Autodesk Fusion 360 part; units mm, degrees
(part 2 of 4)
sketch "스케치3" plane through (0, 0, 0) normal (0, 0, 1) x (1, 0, 0)
  line L0 (5.08, 57.675) -> (15.18, 57.675)
  line L1 (15.18, 57.675) -> (15.18, 47.575)
  line L2 (15.18, 47.575) -> (5.08, 47.575)
  line L3 (5.08, 47.575) -> (5.08, 57.675)
  line L4 (10.13, 57.675) -> (10.13, 47.575) construction
  line L5 (15.18, 52.625) -> (5.08, 52.625) construction
  line L6 (5.08, 53.975) -> (5.08, 51.275) construction
  line L7 (15.18, 53.975) -> (15.18, 51.275) construction
  line L8 (8.78, 57.675) -> (11.48, 57.675) construction
  line L9 (8.78, 47.575) -> (11.48, 47.575) construction
  line L10 (8.78, 57.675) -> (9.13, 56.625)
  line L11 (9.13, 56.625) -> (11.13, 56.625)
  line L12 (11.13, 56.625) -> (11.48, 57.675)
  line L13 (11.48, 47.575) -> (11.13, 48.625)
  line L14 (11.13, 48.625) -> (9.13, 48.625)
  line L15 (9.13, 48.625) -> (8.78, 47.575)
  line L16 (5.08, 51.275) -> (6.13, 51.625)
  line L17 (6.13, 51.625) -> (6.13, 53.625)
  line L18 (6.13, 53.625) -> (5.08, 53.975)
  line L19 (15.18, 53.975) -> (14.13, 53.625)
  line L20 (14.13, 53.625) -> (14.13, 51.625)
  line L21 (14.13, 51.625) -> (15.18, 51.275)
  line L22 (6.13, 53.625) -> (5.08, 53.625) construction
  line L23 (11.13, 56.625) -> (11.13, 57.675) construction
  line L24 (9.13, 48.625) -> (9.13, 47.575) construction
  line L25 (14.13, 51.625) -> (15.18, 51.625) construction
  circle A0 centre (10.13, 52.625) radius 5.05 construction
  line L26 (19.78, 51.625) -> (19.78, 53.625)
  line L27 (18.73, 53.975) -> (18.73, 51.275)
  line L28 (22.43, 47.575) -> (25.13, 47.575)
  line L29 (19.78, 53.625) -> (18.73, 53.625) construction
  line L30 (27.78, 51.625) -> (28.83, 51.275)
  line L31 (18.73, 51.275) -> (19.78, 51.625)
  line L32 (24.78, 56.625) -> (24.78, 57.675) construction
  line L33 (27.78, 53.625) -> (27.78, 51.625)
  line L34 (24.78, 48.625) -> (22.78, 48.625)
  line L35 (28.83, 53.975) -> (27.78, 53.625)
  line L36 (24.78, 56.625) -> (25.13, 57.675)
  line L37 (22.43, 57.675) -> (22.78, 56.625)
  line L38 (28.83, 52.625) -> (18.73, 52.625) construction
  line L39 (28.83, 53.975) -> (28.83, 51.275)
  line L40 (22.78, 48.625) -> (22.43, 47.575)
  line L41 (22.78, 48.625) -> (22.78, 47.575) construction
  line L42 (27.78, 51.625) -> (28.83, 51.625) construction
  line L43 (22.43, 57.675) -> (25.13, 57.675)
  line L44 (25.13, 47.575) -> (24.78, 48.625)
  line L45 (19.78, 53.625) -> (18.73, 53.975)
  line L46 (23.78, 57.675) -> (23.78, 47.575) construction
  line L47 (22.78, 56.625) -> (24.78, 56.625)
  circle A1 centre (23.78, 52.625) radius 5.05 construction
  line L48 (39.07, 56.625) -> (39.42, 57.675)
  line L49 (37.07, 48.625) -> (37.07, 47.575) construction
  line L50 (33.02, 53.975) -> (33.02, 51.275)
  line L51 (36.72, 57.675) -> (37.07, 56.625)
  line L52 (36.72, 57.675) -> (39.42, 57.675)
  line L53 (38.07, 57.675) -> (38.07, 47.575) construction
  line L54 (34.07, 51.625) -> (34.07, 53.625)
  line L55 (37.07, 48.625) -> (36.72, 47.575)
  line L56 (37.07, 56.625) -> (39.07, 56.625)
  line L57 (34.07, 53.625) -> (33.02, 53.975)
  line L58 (33.02, 51.275) -> (34.07, 51.625)
  line L59 (39.07, 48.625) -> (37.07, 48.625)
  line L60 (39.42, 47.575) -> (39.07, 48.625)
  line L61 (36.72, 47.575) -> (39.42, 47.575)
  line L62 (34.07, 53.625) -> (33.02, 53.625) construction
  line L63 (39.07, 56.625) -> (39.07, 57.675) construction
  line L64 (42.07, 51.625) -> (43.12, 51.625) construction
  line L65 (43.12, 52.625) -> (33.02, 52.625) construction
  line L66 (42.07, 51.625) -> (43.12, 51.275)
  line L67 (43.12, 53.975) -> (43.12, 51.275)
  circle A2 centre (38.07, 52.625) radius 5.05 construction
  line L68 (42.07, 53.625) -> (42.07, 51.625)
  line L69 (43.12, 53.975) -> (42.07, 53.625)
  line L70 (53.04, 56.625) -> (53.39, 57.675)
  line L71 (51.04, 48.625) -> (51.04, 47.575) construction
  line L72 (46.99, 53.975) -> (46.99, 51.275)
  line L73 (50.69, 57.675) -> (51.04, 56.625)
  line L74 (50.69, 57.675) -> (53.39, 57.675)
  line L75 (52.04, 57.675) -> (52.04, 47.575) construction
  line L76 (48.04, 51.625) -> (48.04, 53.625)
  line L77 (51.04, 48.625) -> (50.69, 47.575)
  line L78 (51.04, 56.625) -> (53.04, 56.625)
  line L79 (48.04, 53.625) -> (46.99, 53.975)
  line L80 (46.99, 51.275) -> (48.04, 51.625)
  line L81 (53.04, 48.625) -> (51.04, 48.625)
  line L82 (53.39, 47.575) -> (53.04, 48.625)
  line L83 (50.69, 47.575) -> (53.39, 47.575)
  line L84 (48.04, 53.625) -> (46.99, 53.625) construction
  line L85 (53.04, 56.625) -> (53.04, 57.675) construction
  line L86 (56.04, 51.625) -> (57.09, 51.625) construction
  line L87 (57.09, 52.625) -> (46.99, 52.625) construction
  line L88 (56.04, 51.625) -> (57.09, 51.275)
  line L89 (57.09, 53.975) -> (57.09, 51.275)
  circle A3 centre (52.04, 52.625) radius 5.05 construction
  line L90 (56.04, 53.625) -> (56.04, 51.625)
  line L91 (57.09, 53.975) -> (56.04, 53.625)
  line L92 (67.01, 56.625) -> (67.36, 57.675)
  line L93 (65.01, 48.625) -> (65.01, 47.575) construction
  line L94 (60.96, 53.975) -> (60.96, 51.275)
  line L95 (64.66, 57.675) -> (65.01, 56.625)
  line L96 (64.66, 57.675) -> (67.36, 57.675)
  line L97 (66.01, 57.675) -> (66.01, 47.575) construction
  line L98 (62.01, 51.625) -> (62.01, 53.625)
  line L99 (65.01, 48.625) -> (64.66, 47.575)
  line L100 (65.01, 56.625) -> (67.01, 56.625)
  line L101 (62.01, 53.625) -> (60.96, 53.975)
  line L102 (60.96, 51.275) -> (62.01, 51.625)
  line L103 (67.01, 48.625) -> (65.01, 48.625)
  line L104 (67.36, 47.575) -> (67.01, 48.625)
  line L105 (64.66, 47.575) -> (67.36, 47.575)
  line L106 (62.01, 53.625) -> (60.96, 53.625) construction
  line L107 (67.01, 56.625) -> (67.01, 57.675) construction
  line L108 (70.01, 51.625) -> (71.06, 51.625) construction
  line L109 (71.06, 52.625) -> (60.96, 52.625) construction
  line L110 (70.01, 51.625) -> (71.06, 51.275)
  line L111 (71.06, 53.975) -> (71.06, 51.275)
  circle A4 centre (66.01, 52.625) radius 5.05 construction
  line L112 (70.01, 53.625) -> (70.01, 51.625)
  line L113 (71.06, 53.975) -> (70.01, 53.625)
  line L114 (80.98, 56.625) -> (81.33, 57.675)
  line L115 (78.98, 48.625) -> (78.98, 47.575) construction
  line L116 (74.93, 53.975) -> (74.93, 51.275)
  line L117 (78.63, 57.675) -> (78.98, 56.625)
  line L118 (78.63, 57.675) -> (81.33, 57.675)
  line L119 (79.98, 57.675) -> (79.98, 47.575) construction
  line L120 (75.98, 51.625) -> (75.98, 53.625)
  line L121 (78.98, 48.625) -> (78.63, 47.575)
  line L122 (78.98, 56.625) -> (80.98, 56.625)
  line L123 (75.98, 53.625) -> (74.93, 53.975)
  line L124 (74.93, 51.275) -> (75.98, 51.625)
  line L125 (80.98, 48.625) -> (78.98, 48.625)
  line L126 (81.33, 47.575) -> (80.98, 48.625)
  line L127 (78.63, 47.575) -> (81.33, 47.575)
  line L128 (75.98, 53.625) -> (74.93, 53.625) construction
  line L129 (80.98, 56.625) -> (80.98, 57.675) construction
  line L130 (83.98, 51.625) -> (85.03, 51.625) construction
  line L131 (85.03, 52.625) -> (74.93, 52.625) construction
  line L132 (83.98, 51.625) -> (85.03, 51.275)
  line L133 (85.03, 53.975) -> (85.03, 51.275)
  circle A5 centre (79.98, 52.625) radius 5.05 construction
  line L134 (83.98, 53.625) -> (83.98, 51.625)
  line L135 (85.03, 53.975) -> (83.98, 53.625)
  line L136 (94.95, 56.625) -> (95.3, 57.675)
  line L137 (92.95, 48.625) -> (92.95, 47.575) construction
  line L138 (88.9, 53.975) -> (88.9, 51.275)
  line L139 (92.6, 57.675) -> (92.95, 56.625)
  line L140 (92.6, 57.675) -> (95.3, 57.675)
  line L141 (93.95, 57.675) -> (93.95, 47.575) construction
  line L142 (89.95, 51.625) -> (89.95, 53.625)
  line L143 (92.95, 48.625) -> (92.6, 47.575)
  line L144 (92.95, 56.625) -> (94.95, 56.625)
  line L145 (89.95, 53.625) -> (88.9, 53.975)
  line L146 (88.9, 51.275) -> (89.95, 51.625)
  line L147 (94.95, 48.625) -> (92.95, 48.625)
  line L148 (95.3, 47.575) -> (94.95, 48.625)
  line L149 (92.6, 47.575) -> (95.3, 47.575)
  line L150 (89.95, 53.625) -> (88.9, 53.625) construction
  line L151 (94.95, 56.625) -> (94.95, 57.675) construction
  line L152 (97.95, 51.625) -> (99, 51.625) construction
  line L153 (99, 52.625) -> (88.9, 52.625) construction
  line L154 (97.95, 51.625) -> (99, 51.275)
  line L155 (99, 53.975) -> (99, 51.275)
  circle A6 centre (93.95, 52.625) radius 5.05 construction
  line L156 (97.95, 53.625) -> (97.95, 51.625)
  line L157 (99, 53.975) -> (97.95, 53.625)
  line L158 (108.92, 56.625) -> (109.27, 57.675)
  line L159 (106.92, 48.625) -> (106.92, 47.575) construction
  line L160 (102.87, 53.975) -> (102.87, 51.275)
  line L161 (106.57, 57.675) -> (106.92, 56.625)
  line L162 (106.57, 57.675) -> (109.27, 57.675)
  line L163 (107.92, 57.675) -> (107.92, 47.575) construction
  line L164 (103.92, 51.625) -> (103.92, 53.625)
  line L165 (106.92, 48.625) -> (106.57, 47.575)
  line L166 (106.92, 56.625) -> (108.92, 56.625)
  line L167 (103.92, 53.625) -> (102.87, 53.975)
  line L168 (102.87, 51.275) -> (103.92, 51.625)
  line L169 (108.92, 48.625) -> (106.92, 48.625)
  line L170 (109.27, 47.575) -> (108.92, 48.625)
  line L171 (106.57, 47.575) -> (109.27, 47.575)
  line L172 (103.92, 53.625) -> (102.87, 53.625) construction
  line L173 (108.92, 56.625) -> (108.92, 57.675) construction
  line L174 (111.92, 51.625) -> (112.97, 51.625) construction
  line L175 (112.97, 52.625) -> (102.87, 52.625) construction
  line L176 (111.92, 51.625) -> (112.97, 51.275)
  line L177 (112.97, 53.975) -> (112.97, 51.275)
  circle A7 centre (107.92, 52.625) radius 5.05 construction
  line L178 (111.92, 53.625) -> (111.92, 51.625)
  line L179 (112.97, 53.975) -> (111.92, 53.625)
  line L180 (122.89, 56.625) -> (123.24, 57.675)
  line L181 (120.89, 48.625) -> (120.89, 47.575) construction
  line L182 (116.84, 53.975) -> (116.84, 51.275)
  line L183 (120.54, 57.675) -> (120.89, 56.625)
  line L184 (120.54, 57.675) -> (123.24, 57.675)
  line L185 (121.89, 57.675) -> (121.89, 47.575) construction
  line L186 (117.89, 51.625) -> (117.89, 53.625)
  line L187 (120.89, 48.625) -> (120.54, 47.575)
  line L188 (120.89, 56.625) -> (122.89, 56.625)
  line L189 (117.89, 53.625) -> (116.84, 53.975)
  line L190 (116.84, 51.275) -> (117.89, 51.625)
  line L191 (122.89, 48.625) -> (120.89, 48.625)
  line L192 (123.24, 47.575) -> (122.89, 48.625)
  line L193 (120.54, 47.575) -> (123.24, 47.575)
  line L194 (117.89, 53.625) -> (116.84, 53.625) construction
  line L195 (122.89, 56.625) -> (122.89, 57.675) construction
  line L196 (125.89, 51.625) -> (126.94, 51.625) construction
  line L197 (126.94, 52.625) -> (116.84, 52.625) construction
  line L198 (125.89, 51.625) -> (126.94, 51.275)
  line L199 (126.94, 53.975) -> (126.94, 51.275)
  circle A8 centre (121.89, 52.625) radius 5.05 construction
  line L200 (125.89, 53.625) -> (125.89, 51.625)
  line L201 (126.94, 53.975) -> (125.89, 53.625)
  line L202 (136.86, 56.625) -> (137.21, 57.675)
  line L203 (134.86, 48.625) -> (134.86, 47.575) construction
  line L204 (130.81, 53.975) -> (130.81, 51.275)
  line L205 (134.51, 57.675) -> (134.86, 56.625)
  line L206 (134.51, 57.675) -> (137.21, 57.675)
  line L207 (135.86, 57.675) -> (135.86, 47.575) construction
  line L208 (131.86, 51.625) -> (131.86, 53.625)
  line L209 (134.86, 48.625) -> (134.51, 47.575)
  line L210 (134.86, 56.625) -> (136.86, 56.625)
  line L211 (131.86, 53.625) -> (130.81, 53.975)
  line L212 (130.81, 51.275) -> (131.86, 51.625)
  line L213 (136.86, 48.625) -> (134.86, 48.625)
  line L214 (137.21, 47.575) -> (136.86, 48.625)
  line L215 (134.51, 47.575) -> (137.21, 47.575)
  line L216 (131.86, 53.625) -> (130.81, 53.625) construction
  line L217 (136.86, 56.625) -> (136.86, 57.675) construction
  line L218 (139.86, 51.625) -> (140.91, 51.625) construction
  line L219 (140.91, 52.625) -> (130.81, 52.625) construction
  line L220 (139.86, 51.625) -> (140.91, 51.275)
  line L221 (140.91, 53.975) -> (140.91, 51.275)
  circle A9 centre (135.86, 52.625) radius 5.05 construction
  line L222 (139.86, 53.625) -> (139.86, 51.625)
  line L223 (140.91, 53.975) -> (139.86, 53.625)
  circle A10 centre (30.453, 38.655) radius 5.05 construction
  line L224 (29.103, 43.705) -> (29.453, 42.655)
  line L225 (34.453, 37.655) -> (35.503, 37.655) construction
  line L226 (34.453, 39.655) -> (34.453, 37.655)
  line L227 (25.403, 40.005) -> (25.403, 37.305)
  line L228 (31.453, 34.655) -> (29.453, 34.655)
  line L229 (26.453, 37.655) -> (26.453, 39.655)
  line L230 (31.453, 42.655) -> (31.453, 43.705) construction
  line L231 (25.403, 37.305) -> (26.453, 37.655)
  line L232 (31.803, 33.605) -> (31.453, 34.655)
  line L233 (29.453, 34.655) -> (29.453, 33.605) construction
  line L234 (35.503, 40.005) -> (35.503, 37.305)
  line L235 (29.103, 43.705) -> (31.803, 43.705)
  line L236 (35.503, 38.655) -> (25.403, 38.655) construction
  line L237 (29.453, 34.655) -> (29.103, 33.605)
  line L238 (30.453, 43.705) -> (30.453, 33.605) construction
  line L239 (34.453, 37.655) -> (35.503, 37.305)
  line L240 (35.503, 40.005) -> (34.453, 39.655)
  line L241 (29.103, 33.605) -> (31.803, 33.605)
  line L242 (31.453, 42.655) -> (31.803, 43.705)
  line L243 (29.453, 42.655) -> (31.453, 42.655)
  line L244 (26.453, 39.655) -> (25.403, 40.005)
  line L245 (26.453, 39.655) -> (25.403, 39.655) construction
  circle A11 centre (44.423, 38.655) radius 5.05 construction
  line L246 (43.073, 43.705) -> (43.423, 42.655)
  line L247 (48.423, 37.655) -> (49.473, 37.655) construction
  line L248 (48.423, 39.655) -> (48.423, 37.655)
  line L249 (39.373, 40.005) -> (39.373, 37.305)
  line L250 (45.423, 34.655) -> (43.423, 34.655)
  line L251 (40.423, 37.655) -> (40.423, 39.655)
  line L252 (45.423, 42.655) -> (45.423, 43.705) construction
  line L253 (39.373, 37.305) -> (40.423, 37.655)
  line L254 (45.773, 33.605) -> (45.423, 34.655)
  line L255 (43.423, 34.655) -> (43.423, 33.605) construction
  line L256 (49.473, 40.005) -> (49.473, 37.305)
  line L257 (43.073, 43.705) -> (45.773, 43.705)
  line L258 (49.473, 38.655) -> (39.373, 38.655) construction
  line L259 (43.423, 34.655) -> (43.073, 33.605)
  line L260 (44.423, 43.705) -> (44.423, 33.605) construction
  line L261 (48.423, 37.655) -> (49.473, 37.305)
  line L262 (49.473, 40.005) -> (48.423, 39.655)
  line L263 (43.073, 33.605) -> (45.773, 33.605)
  line L264 (45.423, 42.655) -> (45.773, 43.705)
  line L265 (43.423, 42.655) -> (45.423, 42.655)
  line L266 (40.423, 39.655) -> (39.373, 40.005)
  line L267 (40.423, 39.655) -> (39.373, 39.655) construction
  circle A12 centre (58.393, 38.655) radius 5.05 construction
  line L268 (57.043, 43.705) -> (57.393, 42.655)
  line L269 (62.393, 37.655) -> (63.443, 37.655) construction
  line L270 (62.393, 39.655) -> (62.393, 37.655)
  line L271 (53.343, 40.005) -> (53.343, 37.305)
  line L272 (59.393, 34.655) -> (57.393, 34.655)
  line L273 (54.393, 37.655) -> (54.393, 39.655)
  line L274 (59.393, 42.655) -> (59.393, 43.705) construction
  line L275 (53.343, 37.305) -> (54.393, 37.655)
  line L276 (59.743, 33.605) -> (59.393, 34.655)
  line L277 (57.393, 34.655) -> (57.393, 33.605) construction
  line L278 (63.443, 40.005) -> (63.443, 37.305)
  line L279 (57.043, 43.705) -> (59.743, 43.705)
  line L280 (63.443, 38.655) -> (53.343, 38.655) construction
  line L281 (57.393, 34.655) -> (57.043, 33.605)
  line L282 (58.393, 43.705) -> (58.393, 33.605) construction
  line L283 (62.393, 37.655) -> (63.443, 37.305)
  line L284 (63.443, 40.005) -> (62.393, 39.655)
  line L285 (57.043, 33.605) -> (59.743, 33.605)
  line L286 (59.393, 42.655) -> (59.743, 43.705)
  line L287 (57.393, 42.655) -> (59.393, 42.655)
  line L288 (54.393, 39.655) -> (53.343, 40.005)
  line L289 (54.393, 39.655) -> (53.343, 39.655) construction
  circle A13 centre (72.363, 38.655) radius 5.05 construction
  line L290 (71.013, 43.705) -> (71.363, 42.655)
  line L291 (76.363, 37.655) -> (77.413, 37.655) construction
  line L292 (76.363, 39.655) -> (76.363, 37.655)
  line L293 (67.313, 40.005) -> (67.313, 37.305)
  line L294 (73.363, 34.655) -> (71.363, 34.655)
  line L295 (68.363, 37.655) -> (68.363, 39.655)
  line L296 (73.363, 42.655) -> (73.363, 43.705) construction
  line L297 (67.313, 37.305) -> (68.363, 37.655)
  line L298 (73.713, 33.605) -> (73.363, 34.655)
  line L299 (71.363, 34.655) -> (71.363, 33.605) construction
  line L300 (77.413, 40.005) -> (77.413, 37.305)
  line L301 (71.013, 43.705) -> (73.713, 43.705)
  line L302 (77.413, 38.655) -> (67.313, 38.655) construction
  line L303 (71.363, 34.655) -> (71.013, 33.605)
  line L304 (72.363, 43.705) -> (72.363, 33.605) construction
  line L305 (76.363, 37.655) -> (77.413, 37.305)
  line L306 (77.413, 40.005) -> (76.363, 39.655)
  line L307 (71.013, 33.605) -> (73.713, 33.605)
  line L308 (73.363, 42.655) -> (73.713, 43.705)
  line L309 (71.363, 42.655) -> (73.363, 42.655)
  line L310 (68.363, 39.655) -> (67.313, 40.005)
  line L311 (68.363, 39.655) -> (67.313, 39.655) construction
  circle A14 centre (16.483, 38.655) radius 5.05 construction
  line L312 (15.133, 43.705) -> (15.483, 42.655)
  line L313 (20.483, 37.655) -> (21.533, 37.655) construction
  line L314 (20.483, 39.655) -> (20.483, 37.655)
  line L315 (11.433, 40.005) -> (11.433, 37.305)
  line L316 (17.483, 34.655) -> (15.483, 34.655)
  line L317 (12.483, 37.655) -> (12.483, 39.655)
  line L318 (17.483, 42.655) -> (17.483, 43.705) construction
  line L319 (11.433, 37.305) -> (12.483, 37.655)
  line L320 (17.833, 33.605) -> (17.483, 34.655)
  line L321 (15.483, 34.655) -> (15.483, 33.605) construction
  line L322 (21.533, 40.005) -> (21.533, 37.305)
  line L323 (15.133, 43.705) -> (17.833, 43.705)
  line L324 (21.533, 38.655) -> (11.433, 38.655) construction
  line L325 (15.483, 34.655) -> (15.133, 33.605)
  line L326 (16.483, 43.705) -> (16.483, 33.605) construction
  line L327 (20.483, 37.655) -> (21.533, 37.305)
  line L328 (21.533, 40.005) -> (20.483, 39.655)
  line L329 (15.133, 33.605) -> (17.833, 33.605)
  line L330 (17.483, 42.655) -> (17.833, 43.705)
  line L331 (15.483, 42.655) -> (17.483, 42.655)
  line L332 (12.483, 39.655) -> (11.433, 40.005)
  line L333 (12.483, 39.655) -> (11.433, 39.655) construction
  circle A15 centre (86.333, 38.655) radius 5.05 construction
  line L334 (84.983, 43.705) -> (85.333, 42.655)
  line L335 (90.333, 37.655) -> (91.383, 37.655) construction
  line L336 (90.333, 39.655) -> (90.333, 37.655)
  line L337 (81.283, 40.005) -> (81.283, 37.305)
  line L338 (87.333, 34.655) -> (85.333, 34.655)
  line L339 (82.333, 37.655) -> (82.333, 39.655)
  line L340 (87.333, 42.655) -> (87.333, 43.705) construction
  line L341 (81.283, 37.305) -> (82.333, 37.655)
  line L342 (87.683, 33.605) -> (87.333, 34.655)
  line L343 (85.333, 34.655) -> (85.333, 33.605) construction
  line L344 (91.383, 40.005) -> (91.383, 37.305)
  line L345 (84.983, 43.705) -> (87.683, 43.705)
  line L346 (91.383, 38.655) -> (81.283, 38.655) construction
  line L347 (85.333, 34.655) -> (84.983, 33.605)
  line L348 (86.333, 43.705) -> (86.333, 33.605) construction
  line L349 (90.333, 37.655) -> (91.383, 37.305)
  line L350 (91.383, 40.005) -> (90.333, 39.655)
  line L351 (84.983, 33.605) -> (87.683, 33.605)
  line L352 (87.333, 42.655) -> (87.683, 43.705)
  line L353 (85.333, 42.655) -> (87.333, 42.655)
  line L354 (82.333, 39.655) -> (81.283, 40.005)
  line L355 (82.333, 39.655) -> (81.283, 39.655) construction
  circle A16 centre (100.303, 38.655) radius 5.05 construction
  line L356 (98.953, 43.705) -> (99.303, 42.655)
  line L357 (104.303, 37.655) -> (105.353, 37.655) construction
  line L358 (104.303, 39.655) -> (104.303, 37.655)
  line L359 (95.253, 40.005) -> (95.253, 37.305)
  line L360 (101.303, 34.655) -> (99.303, 34.655)
  line L361 (96.303, 37.655) -> (96.303, 39.655)
  line L362 (101.303, 42.655) -> (101.303, 43.705) construction
  line L363 (95.253, 37.305) -> (96.303, 37.655)
  line L364 (101.653, 33.605) -> (101.303, 34.655)
  line L365 (99.303, 34.655) -> (99.303, 33.605) construction
  line L366 (105.353, 40.005) -> (105.353, 37.305)
  line L367 (98.953, 43.705) -> (101.653, 43.705)
  line L368 (105.353, 38.655) -> (95.253, 38.655) construction
  line L369 (99.303, 34.655) -> (98.953, 33.605)
  line L370 (100.303, 43.705) -> (100.303, 33.605) construction
  line L371 (104.303, 37.655) -> (105.353, 37.305)
  line L372 (105.353, 40.005) -> (104.303, 39.655)
  line L373 (98.953, 33.605) -> (101.653, 33.605)
  line L374 (101.303, 42.655) -> (101.653, 43.705)
  line L375 (99.303, 42.655) -> (101.303, 42.655)
  line L376 (96.303, 39.655) -> (95.253, 40.005)
  line L377 (96.303, 39.655) -> (95.253, 39.655) construction
  circle A17 centre (114.273, 38.655) radius 5.05 construction
  line L378 (112.923, 43.705) -> (113.273, 42.655)
  line L379 (118.273, 37.655) -> (119.323, 37.655) construction
  line L380 (118.273, 39.655) -> (118.273, 37.655)
  line L381 (109.223, 40.005) -> (109.223, 37.305)
  line L382 (115.273, 34.655) -> (113.273, 34.655)
  line L383 (110.273, 37.655) -> (110.273, 39.655)
  line L384 (115.273, 42.655) -> (115.273, 43.705) construction
  line L385 (109.223, 37.305) -> (110.273, 37.655)
  line L386 (115.623, 33.605) -> (115.273, 34.655)
  line L387 (113.273, 34.655) -> (113.273, 33.605) construction
  line L388 (119.323, 40.005) -> (119.323, 37.305)
  line L389 (112.923, 43.705) -> (115.623, 43.705)
  line L390 (119.323, 38.655) -> (109.223, 38.655) construction
  line L391 (113.273, 34.655) -> (112.923, 33.605)
  line L392 (114.273, 43.705) -> (114.273, 33.605) construction
  line L393 (118.273, 37.655) -> (119.323, 37.305)
  line L394 (119.323, 40.005) -> (118.273, 39.655)
  line L395 (112.923, 33.605) -> (115.623, 33.605)
  line L396 (115.273, 42.655) -> (115.623, 43.705)
  line L397 (113.273, 42.655) -> (115.273, 42.655)
  line L398 (110.273, 39.655) -> (109.223, 40.005)
  line L399 (110.273, 39.655) -> (109.223, 39.655) construction
  circle A18 centre (128.243, 38.655) radius 5.05 construction
  line L400 (126.893, 43.705) -> (127.243, 42.655)
  line L401 (132.243, 37.655) -> (133.293, 37.655) construction
  line L402 (132.243, 39.655) -> (132.243, 37.655)
  line L403 (123.193, 40.005) -> (123.193, 37.305)
  line L404 (129.243, 34.655) -> (127.243, 34.655)
  line L405 (124.243, 37.655) -> (124.243, 39.655)
  line L406 (129.243, 42.655) -> (129.243, 43.705) construction
  line L407 (123.193, 37.305) -> (124.243, 37.655)
  line L408 (129.593, 33.605) -> (129.243, 34.655)
  line L409 (127.243, 34.655) -> (127.243, 33.605) construction
  line L410 (133.293, 40.005) -> (133.293, 37.305)
  line L411 (126.893, 43.705) -> (129.593, 43.705)
  line L412 (133.293, 38.655) -> (123.193, 38.655) construction
  line L413 (127.243, 34.655) -> (126.893, 33.605)
  line L414 (128.243, 43.705) -> (128.243, 33.605) construction
  line L415 (132.243, 37.655) -> (133.293, 37.305)
  line L416 (133.293, 40.005) -> (132.243, 39.655)
  line L417 (126.893, 33.605) -> (129.593, 33.605)
  line L418 (129.243, 42.655) -> (129.593, 43.705)
  line L419 (127.243, 42.655) -> (129.243, 42.655)
  line L420 (124.243, 39.655) -> (123.193, 40.005)
  line L421 (124.243, 39.655) -> (123.193, 39.655) construction
  circle A19 centre (142.213, 38.655) radius 5.05 construction
  line L422 (140.863, 43.705) -> (141.213, 42.655)
  line L423 (146.213, 37.655) -> (147.263, 37.655) construction
  line L424 (146.213, 39.655) -> (146.213, 37.655)
  line L425 (137.163, 40.005) -> (137.163, 37.305)
  line L426 (143.213, 34.655) -> (141.213, 34.655)
  line L427 (138.213, 37.655) -> (138.213, 39.655)
  line L428 (143.213, 42.655) -> (143.213, 43.705) construction
  line L429 (137.163, 37.305) -> (138.213, 37.655)
  line L430 (143.563, 33.605) -> (143.213, 34.655)
  line L431 (141.213, 34.655) -> (141.213, 33.605) construction
  line L432 (147.263, 40.005) -> (147.263, 37.305)
  line L433 (140.863, 43.705) -> (143.563, 43.705)
  line L434 (147.263, 38.655) -> (137.163, 38.655) construction
  line L435 (141.213, 34.655) -> (140.863, 33.605)
  line L436 (142.213, 43.705) -> (142.213, 33.605) construction
  line L437 (146.213, 37.655) -> (147.263, 37.305)
  line L438 (147.263, 40.005) -> (146.213, 39.655)
  line L439 (140.863, 33.605) -> (143.563, 33.605)
  line L440 (143.213, 42.655) -> (143.563, 43.705)
  line L441 (141.213, 42.655) -> (143.213, 42.655)
  line L442 (138.213, 39.655) -> (137.163, 40.005)
  line L443 (138.213, 39.655) -> (137.163, 39.655) construction
  circle A20 centre (16.483, 38.655) radius 5.05
  circle A21 centre (30.453, 38.655) radius 5.05
  circle A22 centre (44.423, 38.655) radius 5.05
  circle A23 centre (58.393, 38.655) radius 5.05
  circle A24 centre (72.363, 38.655) radius 5.05
  circle A25 centre (86.333, 38.655) radius 5.05
  circle A26 centre (100.303, 38.655) radius 5.05
  circle A27 centre (114.273, 38.655) radius 5.05
  circle A28 centre (128.243, 38.655) radius 5.05
  circle A29 centre (142.213, 38.655) radius 5.05
  line L444 (18.024, 20.05) -> (17.674, 19)
  line L445 (18.024, 20.05) -> (18.024, 19) construction
  line L446 (24.074, 24.05) -> (13.974, 24.05) construction
  line L447 (20.374, 19) -> (20.024, 20.05)
  line L448 (24.074, 25.4) -> (24.074, 22.7)
  line L449 (24.074, 25.4) -> (23.024, 25.05)
  line L450 (20.024, 28.05) -> (20.374, 29.1)
  line L451 (23.024, 25.05) -> (23.024, 23.05)
  line L452 (17.674, 29.1) -> (20.374, 29.1)
  circle A30 centre (19.024, 24.05) radius 5.05 construction
  line L453 (17.674, 19) -> (20.374, 19)
  line L454 (23.024, 23.05) -> (24.074, 23.05) construction
  line L455 (23.024, 23.05) -> (24.074, 22.7)
  line L456 (20.024, 20.05) -> (18.024, 20.05)
  line L457 (20.024, 28.05) -> (20.024, 29.1) construction
  line L458 (15.024, 25.05) -> (13.974, 25.05) construction
  line L459 (17.674, 29.1) -> (18.024, 28.05)
  line L460 (15.024, 25.05) -> (13.974, 25.4)
  line L461 (13.974, 22.7) -> (15.024, 23.05)
  line L462 (18.024, 28.05) -> (20.024, 28.05)
  line L463 (19.024, 29.1) -> (19.024, 19) construction
  line L464 (13.974, 25.4) -> (13.974, 22.7)
  line L465 (15.024, 23.05) -> (15.024, 25.05)
  line L466 (33.274, 20.05) -> (32.924, 19)
  line L467 (38.274, 23.05) -> (39.324, 23.05) construction
  line L468 (39.324, 24.05) -> (29.224, 24.05) construction
  line L469 (29.224, 22.7) -> (30.274, 23.05)
  line L470 (32.924, 19) -> (35.624, 19)
  line L471 (38.274, 23.05) -> (39.324, 22.7)
  line L472 (39.324, 25.4) -> (39.324, 22.7)
  line L473 (39.324, 25.4) -> (38.274, 25.05)
  line L474 (29.224, 25.4) -> (29.224, 22.7)
  line L475 (30.274, 23.05) -> (30.274, 25.05)
  line L476 (35.624, 19) -> (35.274, 20.05)
  line L477 (35.274, 28.05) -> (35.624, 29.1)
  line L478 (35.274, 28.05) -> (35.274, 29.1) construction
  circle A31 centre (34.274, 24.05) radius 5.05 construction
  line L479 (30.274, 25.05) -> (29.224, 25.05) construction
  line L480 (35.274, 20.05) -> (33.274, 20.05)
  line L481 (32.924, 29.1) -> (35.624, 29.1)
  line L482 (33.274, 28.05) -> (35.274, 28.05)
  line L483 (33.274, 20.05) -> (33.274, 19) construction
  line L484 (32.924, 29.1) -> (33.274, 28.05)
  line L485 (34.274, 29.1) -> (34.274, 19) construction
  line L486 (30.274, 25.05) -> (29.224, 25.4)
  line L487 (38.274, 25.05) -> (38.274, 23.05)
  line L488 (53.294, 25.4) -> (53.294, 22.7)
  line L489 (67.264, 24.05) -> (57.164, 24.05) construction
  line L490 (58.214, 25.05) -> (57.164, 25.05) construction
  line L491 (53.294, 25.4) -> (52.244, 25.05)
  line L492 (46.894, 19) -> (49.594, 19)
  line L493 (52.244, 25.05) -> (52.244, 23.05)
  line L494 (61.214, 20.05) -> (60.864, 19)
  line L495 (49.244, 28.05) -> (49.594, 29.1)
  line L496 (61.214, 28.05) -> (63.214, 28.05)
  line L497 (49.594, 19) -> (49.244, 20.05)
  line L498 (52.244, 23.05) -> (53.294, 23.05) construction
  line L499 (46.894, 29.1) -> (49.594, 29.1)
  line L500 (58.214, 25.05) -> (57.164, 25.4)
  line L501 (60.864, 19) -> (63.564, 19)
  line L502 (58.214, 23.05) -> (58.214, 25.05)
  line L503 (49.244, 20.05) -> (47.244, 20.05)
  line L504 (44.244, 25.05) -> (43.194, 25.05) construction
  line L505 (44.244, 23.05) -> (44.244, 25.05)
  line L506 (44.244, 25.05) -> (43.194, 25.4)
  line L507 (63.214, 20.05) -> (61.214, 20.05)
  line L508 (43.194, 22.7) -> (44.244, 23.05)
  line L509 (57.164, 22.7) -> (58.214, 23.05)
  circle A32 centre (48.244, 24.05) radius 5.05 construction
  line L510 (47.244, 28.05) -> (49.244, 28.05)
  line L511 (66.214, 23.05) -> (67.264, 22.7)
  line L512 (47.244, 20.05) -> (46.894, 19)
  line L513 (60.864, 29.1) -> (63.564, 29.1)
  line L514 (66.214, 23.05) -> (67.264, 23.05) construction
  line L515 (63.564, 19) -> (63.214, 20.05)
  line L516 (67.264, 25.4) -> (66.214, 25.05)
  line L517 (57.164, 25.4) -> (57.164, 22.7)
  line L518 (46.894, 29.1) -> (47.244, 28.05)
  circle A33 centre (62.214, 24.05) radius 5.05 construction
  line L519 (47.244, 20.05) -> (47.244, 19) construction
  line L520 (62.214, 29.1) -> (62.214, 19) construction
  line L521 (61.214, 20.05) -> (61.214, 19) construction
  line L522 (43.194, 25.4) -> (43.194, 22.7)
  line L523 (63.214, 28.05) -> (63.214, 29.1) construction
  line L524 (67.264, 25.4) -> (67.264, 22.7)
  line L525 (66.214, 25.05) -> (66.214, 23.05)
  line L526 (48.244, 29.1) -> (48.244, 19) construction
  line L527 (60.864, 29.1) -> (61.214, 28.05)
  line L528 (49.244, 28.05) -> (49.244, 29.1) construction
  line L529 (52.244, 23.05) -> (53.294, 22.7)
  line L530 (53.294, 24.05) -> (43.194, 24.05) construction
  line L531 (63.214, 28.05) -> (63.564, 29.1)
  line L532 (95.204, 25.4) -> (95.204, 22.7)
  line L533 (80.184, 23.05) -> (81.234, 22.7)
  line L534 (80.184, 23.05) -> (81.234, 23.05) construction
  line L535 (81.234, 25.4) -> (81.234, 22.7)
  line L536 (95.204, 24.05) -> (85.104, 24.05) construction
  line L537 (105.474, 19) -> (105.124, 20.05)
  line L538 (86.154, 25.05) -> (85.104, 25.4)
  line L539 (91.154, 28.05) -> (91.504, 29.1)
  circle A34 centre (104.124, 24.05) radius 5.05 construction
  line L540 (91.154, 28.05) -> (91.154, 29.1) construction
  line L541 (100.124, 25.05) -> (99.074, 25.4)
  line L542 (77.184, 28.05) -> (77.534, 29.1)
  line L543 (99.074, 22.7) -> (100.124, 23.05)
  line L544 (105.124, 20.05) -> (103.124, 20.05)
  line L545 (81.234, 25.4) -> (80.184, 25.05)
  line L546 (109.174, 25.4) -> (109.174, 22.7)
  line L547 (89.154, 20.05) -> (88.804, 19)
  line L548 (77.534, 19) -> (77.184, 20.05)
  line L549 (102.774, 29.1) -> (105.474, 29.1)
  line L550 (91.504, 19) -> (91.154, 20.05)
  line L551 (89.154, 20.05) -> (89.154, 19) construction
  line L552 (108.124, 23.05) -> (109.174, 23.05) construction
  line L553 (90.154, 29.1) -> (90.154, 19) construction
  line L554 (74.834, 19) -> (77.534, 19)
  line L555 (105.124, 28.05) -> (105.124, 29.1) construction
  line L556 (85.104, 22.7) -> (86.154, 23.05)
  line L557 (100.124, 25.05) -> (99.074, 25.05) construction
  line L558 (86.154, 25.05) -> (85.104, 25.05) construction
  line L559 (76.184, 29.1) -> (76.184, 19) construction
  line L560 (80.184, 25.05) -> (80.184, 23.05)
  line L561 (77.184, 28.05) -> (77.184, 29.1) construction
  line L562 (103.124, 28.05) -> (105.124, 28.05)
  line L563 (103.124, 20.05) -> (102.774, 19)
  line L564 (99.074, 25.4) -> (99.074, 22.7)
  line L565 (114.094, 25.05) -> (113.044, 25.4)
  line L566 (91.154, 20.05) -> (89.154, 20.05)
  line L567 (86.154, 23.05) -> (86.154, 25.05)
  line L568 (109.174, 25.4) -> (108.124, 25.05)
  circle A35 centre (90.154, 24.05) radius 5.05 construction
  line L569 (72.184, 25.05) -> (71.134, 25.4)
  line L570 (94.154, 25.05) -> (94.154, 23.05)
  line L571 (88.804, 19) -> (91.504, 19)
  line L572 (118.094, 29.1) -> (118.094, 19) construction
  line L573 (94.154, 23.05) -> (95.204, 23.05) construction
  line L574 (71.134, 25.4) -> (71.134, 22.7)
  line L575 (71.134, 22.7) -> (72.184, 23.05)
  line L576 (88.804, 29.1) -> (91.504, 29.1)
  line L577 (123.144, 25.4) -> (122.094, 25.05)
  line L578 (81.234, 24.05) -> (71.134, 24.05) construction
  line L579 (100.124, 23.05) -> (100.124, 25.05)
  line L580 (104.124, 29.1) -> (104.124, 19) construction
  line L581 (74.834, 29.1) -> (77.534, 29.1)
  line L582 (75.184, 20.05) -> (75.184, 19) construction
  line L583 (72.184, 25.05) -> (71.134, 25.05) construction
  line L584 (113.044, 22.7) -> (114.094, 23.05)
  line L585 (108.124, 25.05) -> (108.124, 23.05)
  line L586 (119.094, 28.05) -> (119.444, 29.1)
  line L587 (94.154, 23.05) -> (95.204, 22.7)
  line L588 (75.184, 28.05) -> (77.184, 28.05)
  line L589 (117.094, 28.05) -> (119.094, 28.05)
  line L590 (102.774, 19) -> (105.474, 19)
  line L591 (116.744, 29.1) -> (117.094, 28.05)
  line L592 (74.834, 29.1) -> (75.184, 28.05)
  circle A36 centre (76.184, 24.05) radius 5.05 construction
  line L593 (122.094, 25.05) -> (122.094, 23.05)
  line L594 (77.184, 20.05) -> (75.184, 20.05)
  line L595 (108.124, 23.05) -> (109.174, 22.7)
  line L596 (102.774, 29.1) -> (103.124, 28.05)
  line L597 (122.094, 23.05) -> (123.144, 23.05) construction
  line L598 (72.184, 23.05) -> (72.184, 25.05)
  line L599 (103.124, 20.05) -> (103.124, 19) construction
  line L600 (109.174, 24.05) -> (99.074, 24.05) construction
  line L601 (88.804, 29.1) -> (89.154, 28.05)
  line L602 (85.104, 25.4) -> (85.104, 22.7)
  line L603 (105.124, 28.05) -> (105.474, 29.1)
  line L604 (75.184, 20.05) -> (74.834, 19)
  line L605 (123.144, 25.4) -> (123.144, 22.7)
  line L606 (122.094, 23.05) -> (123.144, 22.7)
  line L607 (114.094, 25.05) -> (113.044, 25.05) construction
  line L608 (119.094, 20.05) -> (117.094, 20.05)
  line L609 (89.154, 28.05) -> (91.154, 28.05)
  line L610 (116.744, 19) -> (119.444, 19)
  line L611 (116.744, 29.1) -> (119.444, 29.1)
  line L612 (117.094, 20.05) -> (117.094, 19) construction
  line L613 (119.444, 19) -> (119.094, 20.05)
  line L614 (95.204, 25.4) -> (94.154, 25.05)
  circle A37 centre (118.094, 24.05) radius 5.05 construction
  line L615 (119.094, 28.05) -> (119.094, 29.1) construction
  line L616 (113.044, 25.4) -> (113.044, 22.7)
  line L617 (117.094, 20.05) -> (116.744, 19)
  line L618 (123.144, 24.05) -> (113.044, 24.05) construction
  line L619 (114.094, 23.05) -> (114.094, 25.05)
  line L620 (81.673, 14.08) -> (83.673, 14.08)
  line L621 (53.673, 6.08) -> (53.323, 5.03)
  circle A38 centre (40.673, 10.08) radius 5.05 construction
  line L622 (12.673, 15.13) -> (12.673, 5.03) construction
  line L623 (26.673, 15.13) -> (26.673, 5.03) construction
  line L624 (78.673, 11.08) -> (77.623, 11.43)
  line L625 (30.673, 9.08) -> (31.723, 8.73)
  line L626 (13.673, 14.08) -> (13.673, 15.13) construction
  line L627 (27.673, 14.08) -> (28.023, 15.13)
  line L628 (39.323, 15.13) -> (39.673, 14.08)
  line L629 (56.023, 5.03) -> (55.673, 6.08)
  line L630 (16.673, 9.08) -> (17.723, 9.08) construction
  line L631 (95.323, 15.13) -> (95.673, 14.08)
  line L632 (55.673, 14.08) -> (55.673, 15.13) construction
  line L633 (96.673, 15.13) -> (96.673, 5.03) construction
  line L634 (72.673, 11.08) -> (72.673, 9.08)
  line L635 (72.673, 9.08) -> (73.723, 8.73)
  line L636 (30.673, 11.08) -> (30.673, 9.08)
  line L637 (59.723, 11.43) -> (58.673, 11.08)
  line L638 (101.723, 11.43) -> (101.723, 8.73)
  line L639 (16.673, 9.08) -> (17.723, 8.73)
  line L640 (41.673, 14.08) -> (41.673, 15.13) construction
  line L641 (87.723, 11.43) -> (87.723, 8.73)
  line L642 (84.023, 5.03) -> (83.673, 6.08)
  line L643 (45.723, 11.43) -> (45.723, 8.73)
  line L644 (27.673, 14.08) -> (27.673, 15.13) construction
  line L645 (36.673, 11.08) -> (35.623, 11.08) construction
  line L646 (58.673, 9.08) -> (59.723, 9.08) construction
  line L647 (31.723, 11.43) -> (30.673, 11.08)
  line L648 (31.723, 11.43) -> (31.723, 8.73)
  line L649 (35.623, 11.43) -> (35.623, 8.73)
  line L650 (30.673, 9.08) -> (31.723, 9.08) construction
  line L651 (55.673, 6.08) -> (53.673, 6.08)
  line L652 (13.673, 14.08) -> (14.023, 15.13)
  line L653 (28.023, 5.03) -> (27.673, 6.08)
  line L654 (68.673, 15.13) -> (68.673, 5.03) construction
  line L655 (69.673, 14.08) -> (70.023, 15.13)
  line L656 (83.673, 14.08) -> (84.023, 15.13)
  line L657 (73.723, 11.43) -> (73.723, 8.73)
  line L658 (17.723, 11.43) -> (17.723, 8.73)
  line L659 (54.673, 15.13) -> (54.673, 5.03) construction
  line L660 (49.623, 11.43) -> (49.623, 8.73)
  line L661 (36.673, 9.08) -> (36.673, 11.08)
  line L662 (97.673, 14.08) -> (97.673, 15.13) construction
  line L663 (11.323, 15.13) -> (11.673, 14.08)
  line L664 (53.323, 15.13) -> (53.673, 14.08)
  line L665 (25.673, 6.08) -> (25.323, 5.03)
  line L666 (55.673, 14.08) -> (56.023, 15.13)
  line L667 (92.673, 9.08) -> (92.673, 11.08)
  line L668 (50.673, 11.08) -> (49.623, 11.08) construction
  line L669 (53.673, 6.08) -> (53.673, 5.03) construction
  line L670 (35.623, 8.73) -> (36.673, 9.08)
  line L671 (45.723, 10.08) -> (35.623, 10.08) construction
  line L672 (25.673, 14.08) -> (27.673, 14.08)
  line L673 (22.673, 11.08) -> (21.623, 11.08) construction
  line L674 (97.673, 6.08) -> (95.673, 6.08)
  line L675 (17.723, 11.43) -> (16.673, 11.08)
  line L676 (25.673, 6.08) -> (25.673, 5.03) construction
  line L677 (21.623, 8.73) -> (22.673, 9.08)
  line L678 (39.323, 5.03) -> (42.023, 5.03)
  line L679 (101.723, 10.08) -> (91.623, 10.08) construction
  line L680 (50.673, 11.08) -> (49.623, 11.43)
  line L681 (16.673, 11.08) -> (16.673, 9.08)
  line L682 (97.673, 14.08) -> (98.023, 15.13)
  line L683 (8.673, 11.08) -> (7.623, 11.08) construction
  line L684 (58.673, 9.08) -> (59.723, 8.73)
  line L685 (25.323, 15.13) -> (25.673, 14.08)
  line L686 (95.673, 6.08) -> (95.673, 5.03) construction
  line L687 (59.723, 10.08) -> (49.623, 10.08) construction
  line L688 (11.673, 6.08) -> (11.323, 5.03)
  line L689 (39.323, 15.13) -> (42.023, 15.13)
  line L690 (7.623, 11.43) -> (7.623, 8.73)
  circle A39 centre (54.673, 10.08) radius 5.05 construction
  line L691 (40.673, 15.13) -> (40.673, 5.03) construction
  line L692 (22.673, 9.08) -> (22.673, 11.08)
  line L693 (63.623, 11.43) -> (63.623, 8.73)
  line L694 (17.723, 10.08) -> (7.623, 10.08) construction
  line L695 (95.323, 15.13) -> (98.023, 15.13)
  line L696 (13.673, 6.08) -> (11.673, 6.08)
  line L697 (86.673, 9.08) -> (87.723, 8.73)
  line L698 (39.673, 6.08) -> (39.323, 5.03)
  circle A40 centre (96.673, 10.08) radius 5.05 construction
  line L699 (44.673, 9.08) -> (45.723, 8.73)
  line L700 (95.673, 6.08) -> (95.323, 5.03)
  line L701 (21.623, 11.43) -> (21.623, 8.73)
  line L702 (95.673, 14.08) -> (97.673, 14.08)
  line L703 (111.673, 14.08) -> (112.023, 15.13)
  line L704 (42.023, 5.03) -> (41.673, 6.08)
  line L705 (39.673, 6.08) -> (39.673, 5.03) construction
  line L706 (59.723, 11.43) -> (59.723, 8.73)
  line L707 (22.673, 11.08) -> (21.623, 11.43)
  line L708 (14.023, 5.03) -> (13.673, 6.08)
  line L709 (8.673, 9.08) -> (8.673, 11.08)
  line L710 (67.323, 15.13) -> (67.673, 14.08)
  line L711 (50.673, 9.08) -> (50.673, 11.08)
  line L712 (64.673, 9.08) -> (64.673, 11.08)
  line L713 (53.323, 5.03) -> (56.023, 5.03)
  line L714 (58.673, 11.08) -> (58.673, 9.08)
  line L715 (25.323, 5.03) -> (28.023, 5.03)
  circle A41 centre (110.673, 10.08) radius 5.05 construction
  line L716 (106.673, 11.08) -> (105.623, 11.43)
  line L717 (8.673, 11.08) -> (7.623, 11.43)
  line L718 (25.323, 15.13) -> (28.023, 15.13)
  line L719 (109.323, 15.13) -> (109.673, 14.08)
  line L720 (44.673, 9.08) -> (45.723, 9.08) construction
  line L721 (112.023, 5.03) -> (111.673, 6.08)
  line L722 (87.723, 11.43) -> (86.673, 11.08)
  line L723 (91.623, 11.43) -> (91.623, 8.73)
  line L724 (44.673, 11.08) -> (44.673, 9.08)
  line L725 (39.673, 14.08) -> (41.673, 14.08)
  line L726 (98.023, 5.03) -> (97.673, 6.08)
  line L727 (114.673, 9.08) -> (115.723, 9.08) construction
  line L728 (101.723, 11.43) -> (100.673, 11.08)
  line L729 (11.673, 6.08) -> (11.673, 5.03) construction
  circle A42 centre (12.673, 10.08) radius 5.05 construction
  line L730 (63.623, 8.73) -> (64.673, 9.08)
  line L731 (86.673, 9.08) -> (87.723, 9.08) construction
  line L732 (11.673, 14.08) -> (13.673, 14.08)
  line L733 (100.673, 9.08) -> (101.723, 8.73)
  line L734 (11.323, 5.03) -> (14.023, 5.03)
  line L735 (87.723, 10.08) -> (77.623, 10.08) construction
  line L736 (67.673, 6.08) -> (67.673, 5.03) construction
  line L737 (31.723, 10.08) -> (21.623, 10.08) construction
  line L738 (100.673, 11.08) -> (100.673, 9.08)
  line L739 (106.673, 9.08) -> (106.673, 11.08)
  line L740 (91.623, 8.73) -> (92.673, 9.08)
  line L741 (41.673, 14.08) -> (42.023, 15.13)
  line L742 (111.673, 14.08) -> (111.673, 15.13) construction
  line L743 (49.623, 8.73) -> (50.673, 9.08)
  line L744 (114.673, 11.08) -> (114.673, 9.08)
  line L745 (109.323, 15.13) -> (112.023, 15.13)
  line L746 (36.673, 11.08) -> (35.623, 11.43)
  line L747 (64.673, 11.08) -> (63.623, 11.08) construction
  circle A43 centre (26.673, 10.08) radius 5.05 construction
  line L748 (95.323, 5.03) -> (98.023, 5.03)
  line L749 (67.673, 6.08) -> (67.323, 5.03)
  line L750 (92.673, 11.08) -> (91.623, 11.08) construction
  line L751 (45.723, 11.43) -> (44.673, 11.08)
  line L752 (109.673, 6.08) -> (109.323, 5.03)
  line L753 (114.673, 9.08) -> (115.723, 8.73)
  line L754 (115.723, 11.43) -> (114.673, 11.08)
  line L755 (92.673, 11.08) -> (91.623, 11.43)
  line L756 (53.323, 15.13) -> (56.023, 15.13)
  line L757 (100.673, 9.08) -> (101.723, 9.08) construction
  line L758 (27.673, 6.08) -> (25.673, 6.08)
  line L759 (64.673, 11.08) -> (63.623, 11.43)
  line L760 (105.623, 11.43) -> (105.623, 8.73)
  line L761 (53.673, 14.08) -> (55.673, 14.08)
  line L762 (7.623, 8.73) -> (8.673, 9.08)
  line L763 (41.673, 6.08) -> (39.673, 6.08)
  circle A44 centre (82.673, 10.08) radius 5.05 construction
  line L764 (115.723, 10.08) -> (105.623, 10.08) construction
  line L765 (106.673, 11.08) -> (105.623, 11.08) construction
  line L766 (111.673, 6.08) -> (109.673, 6.08)
  line L767 (109.673, 14.08) -> (111.673, 14.08)
  line L768 (11.323, 15.13) -> (14.023, 15.13)
  line L769 (109.673, 6.08) -> (109.673, 5.03) construction
  line L770 (110.673, 15.13) -> (110.673, 5.03) construction
  line L771 (105.623, 8.73) -> (106.673, 9.08)
  line L772 (115.723, 11.43) -> (115.723, 8.73)
  line L773 (109.323, 5.03) -> (112.023, 5.03)
  line L774 (77.623, 8.73) -> (78.673, 9.08)
  line L775 (81.673, 6.08) -> (81.673, 5.03) construction
  line L776 (72.673, 9.08) -> (73.723, 9.08) construction
  line L777 (67.323, 15.13) -> (70.023, 15.13)
  line L778 (77.623, 11.43) -> (77.623, 8.73)
  line L779 (86.673, 11.08) -> (86.673, 9.08)
  line L780 (81.323, 15.13) -> (84.023, 15.13)
  line L781 (69.673, 6.08) -> (67.673, 6.08)
  line L782 (67.673, 14.08) -> (69.673, 14.08)
  line L783 (78.673, 9.08) -> (78.673, 11.08)
  line L784 (67.323, 5.03) -> (70.023, 5.03)
  circle A45 centre (68.673, 10.08) radius 5.05 construction
  line L785 (73.723, 10.08) -> (63.623, 10.08) construction
  line L786 (70.023, 5.03) -> (69.673, 6.08)
  line L787 (82.673, 15.13) -> (82.673, 5.03) construction
  line L788 (81.673, 6.08) -> (81.323, 5.03)
  line L789 (83.673, 6.08) -> (81.673, 6.08)
  line L790 (73.723, 11.43) -> (72.673, 11.08)
  line L791 (78.673, 11.08) -> (77.623, 11.08) construction
  line L792 (69.673, 14.08) -> (69.673, 15.13) construction
  line L793 (81.323, 5.03) -> (84.023, 5.03)
  line L794 (81.323, 15.13) -> (81.673, 14.08)
  line L795 (83.673, 14.08) -> (83.673, 15.13) construction
  line L796 (131.064, 20.05) -> (131.064, 19) construction
  line L797 (142.034, 25.05) -> (140.984, 25.05) construction
  line L798 (147.034, 28.05) -> (147.384, 29.1)
  line L799 (137.673, 14.08) -> (139.673, 14.08)
  line L800 (119.623, 11.43) -> (119.623, 8.73)
  line L801 (143.723, 11.43) -> (142.673, 11.08)
  line L802 (137.323, 15.13) -> (140.023, 15.13)
  line L803 (133.623, 8.73) -> (134.673, 9.08)
  line L804 (147.384, 19) -> (147.034, 20.05)
  line L805 (145.034, 20.05) -> (144.684, 19)
  line L806 (147.034, 20.05) -> (145.034, 20.05)
  line L807 (123.673, 6.08) -> (123.673, 5.03) construction
  line L808 (134.673, 9.08) -> (134.673, 11.08)
  line L809 (138.673, 15.13) -> (138.673, 5.03) construction
  line L810 (143.723, 11.43) -> (143.723, 8.73)
  line L811 (127.014, 25.4) -> (127.014, 22.7)
  line L812 (127.014, 22.7) -> (128.064, 23.05)
  line L813 (151.084, 25.4) -> (150.034, 25.05)
  line L814 (145.034, 20.05) -> (145.034, 19) construction
  line L815 (142.673, 9.08) -> (143.723, 8.73)
  line L816 (131.064, 20.05) -> (130.714, 19)
  line L817 (131.064, 28.05) -> (133.064, 28.05)
  line L818 (137.114, 24.05) -> (127.014, 24.05) construction
  line L819 (142.034, 25.05) -> (140.984, 25.4)
  line L820 (144.684, 29.1) -> (147.384, 29.1)
  line L821 (128.064, 25.05) -> (127.014, 25.4)
  line L822 (129.723, 10.08) -> (119.623, 10.08) construction
  line L823 (136.064, 23.05) -> (137.114, 22.7)
  circle A46 centre (124.673, 10.08) radius 5.05 construction
  line L824 (130.714, 29.1) -> (131.064, 28.05)
  line L825 (146.034, 29.1) -> (146.034, 19) construction
  line L826 (140.984, 25.4) -> (140.984, 22.7)
  line L827 (125.673, 6.08) -> (123.673, 6.08)
  line L828 (123.323, 5.03) -> (126.023, 5.03)
  line L829 (128.064, 25.05) -> (127.014, 25.05) construction
  circle A47 centre (146.034, 24.05) radius 5.05 construction
  line L830 (123.323, 15.13) -> (126.023, 15.13)
  line L831 (123.673, 14.08) -> (125.673, 14.08)
  line L832 (128.064, 23.05) -> (128.064, 25.05)
  line L833 (144.684, 19) -> (147.384, 19)
  line L834 (130.714, 19) -> (133.414, 19)
  line L835 (140.984, 22.7) -> (142.034, 23.05)
  circle A48 centre (138.673, 10.08) radius 5.05 construction
  line L836 (142.673, 11.08) -> (142.673, 9.08)
  line L837 (137.323, 15.13) -> (137.673, 14.08)
  line L838 (139.673, 14.08) -> (139.673, 15.13) construction
  line L839 (137.323, 5.03) -> (140.023, 5.03)
  line L840 (150.034, 23.05) -> (151.084, 22.7)
  line L841 (134.673, 11.08) -> (133.623, 11.08) construction
  line L842 (151.084, 24.05) -> (140.984, 24.05) construction
  line L843 (143.723, 10.08) -> (133.623, 10.08) construction
  line L844 (123.323, 15.13) -> (123.673, 14.08)
  line L845 (145.034, 28.05) -> (147.034, 28.05)
  line L846 (150.034, 23.05) -> (151.084, 23.05) construction
  line L847 (119.623, 8.73) -> (120.673, 9.08)
  line L848 (120.673, 9.08) -> (120.673, 11.08)
  line L849 (142.673, 9.08) -> (143.723, 9.08) construction
  line L850 (134.673, 11.08) -> (133.623, 11.43)
  line L851 (120.673, 11.08) -> (119.623, 11.08) construction
  line L852 (147.034, 28.05) -> (147.034, 29.1) construction
  circle A49 centre (132.064, 24.05) radius 5.05 construction
  line L853 (151.084, 25.4) -> (151.084, 22.7)
  line L854 (133.064, 20.05) -> (131.064, 20.05)
  line L855 (137.673, 6.08) -> (137.323, 5.03)
  line L856 (120.673, 11.08) -> (119.623, 11.43)
  line L857 (140.023, 5.03) -> (139.673, 6.08)
  line L858 (133.623, 11.43) -> (133.623, 8.73)
  line L859 (139.673, 14.08) -> (140.023, 15.13)
  line L860 (130.714, 29.1) -> (133.414, 29.1)
  line L861 (137.673, 6.08) -> (137.673, 5.03) construction
  line L862 (144.684, 29.1) -> (145.034, 28.05)
  line L863 (142.034, 23.05) -> (142.034, 25.05)
  line L864 (139.673, 6.08) -> (137.673, 6.08)
  line L865 (123.673, 6.08) -> (123.323, 5.03)
  line L866 (150.034, 25.05) -> (150.034, 23.05)
  line L867 (136.064, 23.05) -> (137.114, 23.05) construction
  line L868 (133.064, 28.05) -> (133.414, 29.1)
  line L869 (128.673, 9.08) -> (129.723, 9.08) construction
  line L870 (133.064, 28.05) -> (133.064, 29.1) construction
  line L871 (128.673, 9.08) -> (129.723, 8.73)
  line L872 (136.064, 25.05) -> (136.064, 23.05)
  line L873 (137.114, 25.4) -> (137.114, 22.7)
  line L874 (129.723, 11.43) -> (129.723, 8.73)
  line L875 (126.023, 5.03) -> (125.673, 6.08)
  line L876 (137.114, 25.4) -> (136.064, 25.05)
  line L877 (133.414, 19) -> (133.064, 20.05)
  line L878 (125.673, 14.08) -> (126.023, 15.13)
  line L879 (132.064, 29.1) -> (132.064, 19) construction
  line L880 (128.673, 11.08) -> (128.673, 9.08)
  line L881 (124.673, 15.13) -> (124.673, 5.03) construction
  line L882 (129.723, 11.43) -> (128.673, 11.08)
  line L883 (125.673, 14.08) -> (125.673, 15.13) construction
  circle A50 centre (12.673, 10.08) radius 5.05
  circle A51 centre (26.673, 10.08) radius 5.05
  circle A52 centre (40.673, 10.08) radius 5.05
  circle A53 centre (54.673, 10.08) radius 5.05
  circle A54 centre (68.673, 10.08) radius 5.05
  circle A55 centre (82.673, 10.08) radius 5.05
  circle A56 centre (96.673, 10.08) radius 5.05
  circle A57 centre (110.673, 10.08) radius 5.05
  circle A58 centre (124.673, 10.08) radius 5.05
  circle A59 centre (138.673, 10.08) radius 5.05
  circle A60 centre (146.034, 24.05) radius 5.05
  circle A61 centre (132.064, 24.05) radius 5.05
  circle A62 centre (118.094, 24.05) radius 5.05
  circle A63 centre (104.124, 24.05) radius 5.05
  circle A64 centre (90.154, 24.05) radius 5.05
  circle A65 centre (76.184, 24.05) radius 5.05
  circle A66 centre (62.214, 24.05) radius 5.05
  circle A67 centre (48.244, 24.05) radius 5.05
  circle A68 centre (34.274, 24.05) radius 5.05
  circle A69 centre (19.024, 24.05) radius 5.05
  point P0 (23.78, 52.625)
  point P1 (38.07, 52.625)
  point P2 (52.04, 52.625)
  point P3 (66.01, 52.625)
  point P4 (79.98, 52.625)
  point P5 (93.95, 52.625)
  point P6 (107.92, 52.625)
  point P7 (121.89, 52.625)
  point P8 (135.86, 52.625)
  point P9 (30.453, 38.655)
  point P10 (44.423, 38.655)
  point P11 (58.393, 38.655)
  point P12 (72.363, 38.655)
  point P13 (86.333, 38.655)
  point P14 (100.303, 38.655)
  point P15 (114.273, 38.655)
  point P16 (128.243, 38.655)
  point P17 (142.213, 38.655)
  point P18 (16.483, 38.655)
  point P19 (30.453, 38.655)
  point P20 (142.213, 38.655)
  point P21 (128.243, 38.655)
  point P22 (114.273, 38.655)
  point P23 (100.303, 38.655)
  point P24 (86.333, 38.655)
  point P25 (72.363, 38.655)
  point P26 (58.393, 38.655)
  point P27 (44.423, 38.655)
  point P28 (19.024, 24.05)
  point P29 (34.274, 24.05)